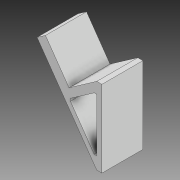
# Autodesk Inventor part: LEDbracket
Saved by Autodesk Inventor 2020 (Build 240168000, 168)
## iProperties
Created: 2021-01-14
Part Number: LEDbracket
Material: Generic
Document SubType Name: Modeling
Designer: DDeGo
Density: 1 g/cm^3
Appearance: Default
Author: DDeGo
Autodesk Inventor part; units mm, degrees
ref_plane "YZ Plane" through (0, 0, 0) normal (1, 0, 0) x (0, 1, 0)
ref_plane "XZ Plane" through (0, 0, 0) normal (0, 1, 0) x (-1, 0, 0)
ref_plane "XY Plane" through (0, 0, 0) normal (0, 0, 1) x (1, 0, 0)
sketch "Sketch1" plane through (0, 0, 0) normal (0, 0, 1) x (1, 0, 0)
  line L0 (0, 0) -> (1, 0)
  line L1 (1, 0) -> (1, 15)
  line L2 (1, 15) -> (0, 15)
  line L3 (0, 15) -> (-5.4094, 11.2123)
  line L4 (-5.4094, 11.2123) -> (-9.998, 17.7655)
  line L5 (-9.998, 17.7655) -> (-11.6363, 16.6184)
  line L6 (-11.6363, 16.6184) -> (0, 0)
  line L7 (-0.5, 12.8187) -> (-5.1333, 9.5745)
  line L8 (-5.1333, 9.5745) -> (-5.1333, 9.0745)
  line L9 (-5.1333, 9.0745) -> (-0.5, 2.4575)
  line L10 (-0.5, 2.4575) -> (0, 2.4575)
  line L11 (0, 2.4575) -> (0, 12.8187)
  line L12 (0, 12.8187) -> (-0.5, 12.8187)
  dimension "d0" = 35
  dimension "d1" = 1
  dimension "d2" = 2
  dimension "d3" = 8
  dimension "d4" = 15
  dimension "d5" = 1
  dimension "d6" = 0.5
  dimension "d7" = 0.5
  dimension "d8" = 0.5
  dimension "d9" = 1
  dimension "d11" = 1.5
  dimension "d12" = 1
  constraints: 26 end point, 6 perpendicular, 4 parallel, 1 horizontal, 1 vertical
  measures "d0" angle of L0 L3
  measures "d1" distance of L1.end L2.end
  measures "d2" distance between parallel lines of L6 L4
  measures "d3" distance of L3.end L4.end
  measures "d4" distance of L0.end L1.end
  measures "d5" distance of L0.start L0.end
  measures "d6" distance of L11.end L7.start
  measures "d7" distance of L7.end L8.end
  measures "d8" distance of L9.end L10.end
  measures "d9" distance between parallel lines of L1 L11
  measures "d11" distance between parallel lines of L3 L7
  measures "d12" distance between parallel lines of L6 L9
extrude "Extrusion1" add sketch "Sketch1" along normal mid plane 8
body "Solid1"
